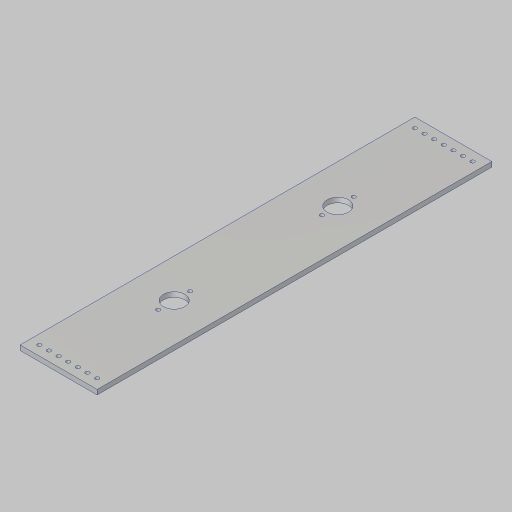
# Autodesk Inventor part: GI - 007
Saved by Autodesk Inventor 2023.5 (Build 275446000, 446)
## iProperties
Created: 2025-01-26
Part Number: GI - 007
Material: Aluminum 6061
Document SubType Name: Modeling
Designer: slick
Density: 2.7 g/cm^3
Appearance: Aluminum - Flat
Mass: 902.825 g
Surface Area: 1159.32 cm^2
Volume: 334.38 cm^3
Author: slick
Autodesk Inventor part; units mm, degrees
ref_plane "YZ Plane" through (0, 0, 0) normal (1, 0, 0) x (0, 1, 0)
ref_plane "XZ Plane" through (0, 0, 0) normal (0, 1, 0) x (-1, 0, 0)
ref_plane "XY Plane" through (0, 0, 0) normal (0, 0, 1) x (1, 0, 0)
sketch "Sketch1" plane through (0, 0, 0) normal (0, 1, 0) x (-1, 0, 0)
  line L0 (-50.8, -260.35) -> (50.8, -260.35)
  line L1 (50.8, -260.35) -> (50.8, 260.35)
  line L2 (50.8, 260.35) -> (-50.8, 260.35)
  line L3 (-50.8, 260.35) -> (-50.8, -260.35)
  line L4 (-50.8, -260.35) -> (50.8, 260.35) construction
  line L5 (50.8, -260.35) -> (-50.8, 260.35) construction
  point P0 (0, 0)
  dimension "d0" = 101.6
  dimension "d1" = 520.7
  constraints: 12 end point, 2 midpoint, 2 parallel, 1 horizontal, 1 perpendicular
  measures "d0" distance of L2.end L1.end
  measures "d1" distance of L1.end L0.end
extrude "Extrusion1" add sketch "Sketch1" along normal blind 6.35
sketch "Sketch2" plane through (0, 6.35, 0) normal (0, 1, 0) x (1, 0, 0)
  circle A0 centre (0, -107.95) radius 14.097
  circle A1 centre (0, 107.95) radius 14.097
  line L0 (0, -107.95) -> (0, 107.95) construction
  circle A2 centre (0, -107.95) radius 63.5 construction
  circle A3 centre (0, 107.95) radius 63.5 construction
  circle A4 centre (-107.4015, 0) radius 57.15 construction
  circle A5 centre (0, 44.5491) radius 14.097
  point P0 (0, 0)
  point P1 (0, 0)
  point P2 (0, -44.45)
  point P3 (0, 44.45)
  dimension "d7" = 127
  dimension "d8" = 127
  dimension "d5" = 28.194
  dimension "d9" = 88.9
  dimension "d10" = 114.3
  dimension "d12" = 152.4991
  constraints: 4 centre point, 4 vertical alignment, 3 coincident, 3 point on line, 2 end point, 2 equal radius, 1 horizontal alignment, 1 midpoint, 1 vertical, 4 other
  measures "d5" diameter of A1
  measures "d9" distance of point (0, 44.45) point (0, -44.45)
  measures "d10" diameter of A4
  measures "d12" distance of A5.centre L0.start
extrude "Extrusion2" cut sketch "Sketch2" against normal blind 6.35 contours A0 | A1
sketch "Sketch3" plane through (0, 6.35, 0) normal (0, 1, 0) x (1, 0, 0)
  line L0 (-50.8, -260.35) -> (50.8, -260.35) projected
  line L1 (-50.8, 260.35) -> (-50.8, -260.35) projected
  line L2 (-50.8, 260.35) -> (-50.8, -260.35) construction
  line L3 (-50.8, 0) -> (50.8, 0) construction
  line L4 (50.8, -260.35) -> (50.8, 260.35) construction
  point P0 (0, 0)
  point P1 (-38.1, -247.65)
  point P2 (-25.4, -247.65)
  point P3 (-12.7, -247.65)
  point P4 (0, -247.65)
  point P5 (12.7, -247.65)
  point P6 (25.4, -247.65)
  point P7 (38.1, -247.65)
  point P8 (-38.1, 247.65)
  point P9 (-25.4, 247.65)
  point P10 (-12.7, 247.65)
  point P11 (0, 247.65)
  point P12 (12.7, 247.65)
  point P13 (25.4, 247.65)
  point P14 (38.1, 247.65)
  dimension "d15" = 12.7
  dimension "d16" = 12.7
  dimension "d19" = 12.7
  constraints: 7 symmetric about line, 2 end point, 2 midpoint, 1 horizontal, 6 other
  measures "d15" distance from line of L0 point (-38.1, -247.65)
  measures "d16" distance from line of L1 point (-38.1, -247.65)
  measures "d19" distance of point (-38.1, -247.65) point (-25.4, -247.65)
hole "Hole1" at (-38.1, 6.35, 247.65) at (-25.4, 6.35, 247.65) at (-12.7, 6.35, 247.65) at (0, 6.35, 247.65) at (12.7, 6.35, 247.65) at (25.4, 6.35, 247.65) at (38.1, 6.35, 247.65) at (38.1, 6.35, -247.65) at (25.4, 6.35, -247.65) at (12.7, 6.35, -247.65) at (0, 6.35, -247.65) at (-12.7, 6.35, -247.65) at (-25.4, 6.35, -247.65) at (-38.1, 6.35, -247.65) direction (0, -1, 0) diameter 5.1054 end through all clearance for "Flat Head Machine Screw (82)" size "#10" standard "Ansi Unified Screw Threads"
sketch "Sketch4" plane through (0, 6.35, 0) normal (0, 1, 0) x (1, 0, 0)
  line L0 (0, -86.9315) -> (0, -128.9685) construction
  line L1 (0, 128.9685) -> (0, 86.9315) construction
  circle A0 centre (-25.4, 247.65) radius 2.5527 projected
  circle A1 centre (0, 247.65) radius 2.5527 projected
  circle A2 centre (25.4, 247.65) radius 2.5527 projected
  circle A3 centre (38.1, -247.65) radius 2.5527 projected
  circle A4 centre (12.7, -247.65) radius 2.5527 projected
  circle A5 centre (-12.7, -247.65) radius 2.5527 projected
  circle A6 centre (-38.1, -247.65) radius 2.5527 projected
  circle A7 centre (-25.4, -247.65) radius 2.5527 projected
  circle A8 centre (0, -247.65) radius 2.5527 projected
  circle A9 centre (25.4, -247.65) radius 2.5527 projected
  circle A10 centre (38.1, 247.65) radius 2.5527 projected
  circle A11 centre (12.7, 247.65) radius 2.5527 projected
  circle A12 centre (-12.7, 247.65) radius 2.5527 projected
  circle A13 centre (-38.1, 247.65) radius 2.5527 projected
  circle A14 centre (0, 107.95) radius 14.097 projected
  circle A15 centre (0, -107.95) radius 14.097 projected
  line L2 (-50.8, 260.35) -> (50.8, 260.35) projected
  line L3 (50.8, 260.35) -> (50.8, -260.35) projected
  line L4 (50.8, -260.35) -> (-50.8, -260.35) projected
  line L5 (-50.8, -260.35) -> (-50.8, 260.35) projected
  point P0 (0, 0)
  dimension "d31" = 42.037
  dimension "d32" = 42.037
  constraints: 4 coincident, 4 end point, 2 midpoint, 2 vertical, 1 vertical alignment
  measures "d31" distance of L1.start L1.end
  measures "d32" distance of L0.start L0.end
hole "Hole2" at (0, 6.35, -128.9685) at (0, 6.35, -86.9315) at (0, 6.35, 86.9315) at (0, 6.35, 128.9685) direction (0, -1, 0) diameter 5.1054 end through all clearance for "Flat Head Machine Screw (82)" size "#10" standard "Ansi Unified Screw Threads"
body "Solid1"
